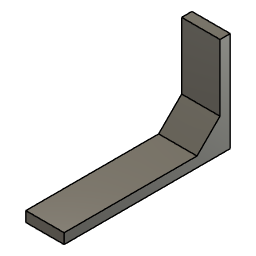
angle_90deg_profile_mount_v1 (Autodesk Fusion 360 design; units mm, degrees)
Autodesk Fusion 360 part; units mm, degrees
box "BoxPrimitive1" add length 65 width 15 height 4 placed x (0, 0, -1) y (-1, 0, 0) z (0, 1, 0) at (0, 0, 0)
sketch "Sketch2" plane through (0, 4, 0) normal (0, 1, 0) x (-1, 0, 0)
  line L0 (0, -65) -> (15, -65)
  line L1 (15, -65) -> (15, 0)
  line L2 (15, 0) -> (0, 0)
  line L3 (0, 0) -> (0, -65)
  line L4 (15, -65) -> (0, -65)
  line L5 (0, -65) -> (0, -61)
  line L6 (0, -61) -> (15, -61)
  line L7 (15, -61) -> (15, -65)
  dimension "d6" = 4
  constraint horizontal L4
  constraint vertical L5
  constraint horizontal L6
  constraint vertical L7
  constraint coincident L3 L5.end
  constraint coincident L0.end L1.start
  measures "d6" distance of L0.start L5.end
extrude "Extrude1" add sketch "Sketch2" along normal blind 35 contours L0 L1 L3 L4 L5 L6 L7
chamfer "Chamfer1" distance 9 angle 45 1 edges at (-7.5, 4, -61)
